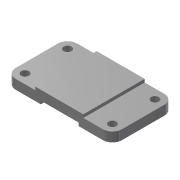
# Autodesk Inventor part: Base Plate
Saved by Autodesk Inventor 2022 Beta2 (Build 260130000, 130) ContinuousBuild 0
## iProperties
Created: 2007-03-01
Part Number: Base Plate
Document SubType Name: Modeling
Designer: MFlayler
Material: Carbon Steel
Mass: 982.528 g
Surface Area: 279.092 cm^2
Volume: 125.163 cm^3
Density: 7.85 g/cm^3
Appearance: Steel
Author: MFlayler
Autodesk Inventor part; units mm, degrees
ref_plane "YZ Plane" through (0, 0, 0) normal (1, 0, 0) x (0, 1, 0)
ref_plane "XZ Plane" through (0, 0, 0) normal (0, 1, 0) x (-1, 0, 0)
sketch "Sketch1" plane through (0, 0, 0) normal (0, 0, 1) x (1, 0, 0)
  line L0 (-67.5, -39) -> (67.5, -39)
  line L1 (67.5, -39) -> (67.5, 39)
  line L2 (67.5, 39) -> (-67.5, 39)
  line L3 (-67.5, 39) -> (-67.5, -39)
  point P0 (0, 0)
  point P1 (-67.5, 0)
  point P2 (0, 39)
  dimension "d0" = 78
  dimension "d1" = 135
  constraints: 8 end point, 2 midpoint, 2 parallel, 1 horizontal, 1 horizontal alignment, 1 perpendicular, 1 vertical alignment
  measures "d0" distance of L2.end L0.start
  measures "d1" distance of L1.end L2.end
extrude "Extrusion1" add sketch "Sketch1" along normal blind 12
sketch "Sketch2" plane through (0, 0, 12) normal (0, 0, 1) x (1, 0, 0)
  line L0 (67.5, -39) -> (-67.5, -39) projected
  line L1 (-67.5, 39) -> (67.5, 39) projected
  line L2 (-30.5, -39) -> (30.5, -39)
  line L3 (30.5, -39) -> (30.5, 39)
  line L4 (30.5, 39) -> (-30.5, 39)
  line L5 (-30.5, 39) -> (-30.5, -39)
  line L6 (0, 54.6) -> (0, -54.6) projected
  line L7 (-95.2, 0) -> (95.2, 0) projected
  dimension "d4" = 61
  constraints: 8 end point, 2 parallel, 2 point on line, 1 horizontal, 1 perpendicular, 1 other
  measures "d4" distance between parallel lines of L3 L5
extrude "Extrusion2" add sketch "Sketch2" along normal blind 4
sketch "Sketch3" plane through (0, 0, 0) normal (0, 0, -1) x (-1, 0, 0)
  line L0 (67.5, -39) -> (-67.5, -39) projected
  line L1 (67.5, 39) -> (67.5, -39) projected
  line L2 (-67.5, 39) -> (67.5, 39) projected
  line L3 (23.5, -39) -> (-24.5, -39)
  line L4 (-24.5, -39) -> (-24.5, 39)
  line L5 (-24.5, 39) -> (23.5, 39)
  line L6 (23.5, 39) -> (23.5, -39)
  dimension "d8" = 48
  dimension "d9" = 44
  constraints: 8 end point, 2 parallel, 2 point on line, 1 horizontal, 1 perpendicular
  measures "d8" distance between parallel lines of L4 L6
  measures "d9" distance between parallel lines of L6 L1
extrude "Extrusion3" cut sketch "Sketch3" against normal blind 4 contours L0 L4 L2 L6
sketch "Sketch4" plane through (0, 0, 12) normal (0, 0, 1) x (1, 0, 0)
  line L0 (67.5, 39) -> (67.5, -39) projected
  line L1 (30.5, 39) -> (67.5, 39) projected
  line L2 (67.5, 0) -> (0.1063, 0) construction
  line L3 (-30.5, -39) -> (-30.5, 39) projected
  line L4 (30.5, -39) -> (-30.5, -39) projected
  line L5 (30.5, 39) -> (30.5, -39) projected
  line L6 (-30.5, 39) -> (30.5, 39) projected
  line L7 (-30.5, -39) -> (-30.5, 39) projected
  line L8 (-67.5, 39) -> (-30.5, 39) projected
  line L9 (-67.5, -39) -> (-67.5, 39) projected
  line L10 (-30.5, -39) -> (-67.5, -39) projected
  line L11 (0, 39) -> (0, 3.4704) construction
  point P0 (55.5, 27)
  point P1 (-55.5, 27)
  point P2 (-55.5, -27)
  point P3 (55.5, -27)
  dimension "d12" = 111
  dimension "d13" = 54
  constraints: 4 end point, 2 midpoint, 2 symmetric about line, 2 vertical alignment, 1 horizontal alignment, 1 parallel, 1 perpendicular
  measures "d12" distance of point (-55.5, 27) point (55.5, 27)
  measures "d13" distance of point (55.5, 27) point (55.5, -27)
hole "Hole1" at (55.5, 27, 12) at (-55.5, 27, 12) at (-55.5, -27, 12) at (55.5, -27, 12) direction (0, 0, -1) diameter 10 depth 12
fillet "Fillet1" radius 12 4 edges at (67.5, 39, 6) (67.5, -39, 6) (-67.5, 39, 6) (-67.5, -39, 6)
ref_plane "Midplane" through (0, -39, 16) normal (1, 0, 0) x (0, 0, -1)
body "Solid1"
